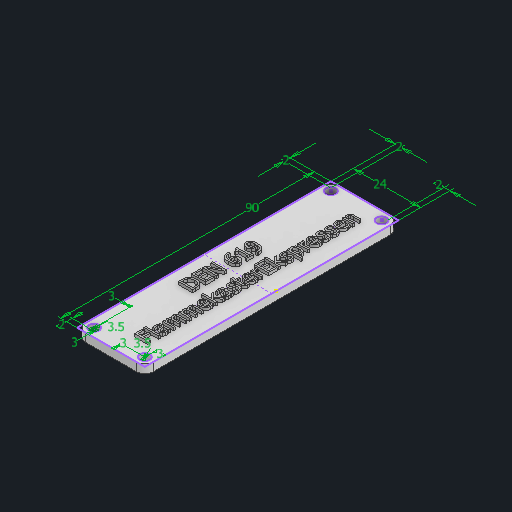
# Autodesk Inventor part: Flammekasterekspressen
Saved by Autodesk Inventor 2026.2 (Build 302298000, 298)
## iProperties
Created: 2026-05-12
Part Number: Flammekasterekspressen
Material: Generic
Document SubType Name: Modeling
Designer: Malthe Sennels
Density: 1 g/cm^3
Appearance: Default
Author: Malthe Sennels
Autodesk Inventor part; units mm, degrees
ref_plane "YZ Plane" through (0, 0, 0) normal (1, 0, 0) x (0, 1, 0)
ref_plane "XZ Plane" through (0, 0, 0) normal (0, 1, 0) x (-1, 0, 0)
ref_plane "XY Plane" through (0, 0, 0) normal (0, 0, 1) x (1, 0, 0)
sketch "Sketch1" plane through (0, 0, 0) normal (0, 1, 0) x (-1, 0, 0)
  line L0 (24.0563, 46.4821) -> (0.0563, 46.4821)
  line L1 (0.0563, 46.4821) -> (0.0563, -43.5179)
  line L2 (0.0563, -43.5179) -> (24.0563, -43.5179)
  line L3 (24.0563, -43.5179) -> (24.0563, 46.4821)
  line L4 (22.0563, 44.4821) -> (22.0563, -41.5179) construction
  line L5 (22.0563, -41.5179) -> (2.0563, -41.5179) construction
  line L6 (2.0563, -41.5179) -> (2.0563, 44.4821) construction
  line L7 (2.0563, 44.4821) -> (22.0563, 44.4821) construction
  circle A0 centre (21.0563, 43.4821) radius 1.75
  circle A1 centre (3.0563, 43.4821) radius 1.75
  line L8 (24.0563, 1.4821) -> (0.0563, 1.4821) construction
  circle A2 centre (21.0563, -40.5179) radius 1.75
  circle A3 centre (3.0563, -40.5179) radius 1.75
  spline S0 degree 2 poles (16.8086, 11.3646) (16.1238, 11.3646) (15.0217, 11.9197) (14.7138, 12.3857) knots 0 0 0 1 2 2 2
  spline S1 degree 2 poles (14.7138, 12.3857) (14.4747, 12.7666) (14.3126, 13.5486) (14.3126, 14.1564) knots 0 0 0 1 2 2 2
  line L9 (14.3126, 14.1564) -> (14.3126, 15.3071)
  line L10 (14.3126, 15.3071) -> (19.3126, 15.3071)
  line L11 (19.3126, 15.3071) -> (19.3126, 14.1685)
  spline S2 degree 2 poles (19.3126, 14.1685) (19.3126, 13.4635) (19.1019, 12.6612) (18.9156, 12.3776) knots 0 0 0 1 2 2 2
  spline S3 degree 2 poles (18.9156, 12.3776) (18.5955, 11.8954) (17.5379, 11.3646) (16.8086, 11.3646) knots 0 0 0 1 2 2 2
  spline S4 degree 2 poles (16.8167, 12.0575) (17.3921, 12.0575) (18.2065, 12.4384) (18.4374, 12.8152) knots 0 0 0 1 2 2 2
  spline S5 degree 2 poles (18.4374, 12.8152) (18.5955, 13.0826) (18.7373, 13.6863) (18.7373, 14.1361) knots 0 0 0 1 2 2 2
  line L12 (18.7373, 14.1361) -> (18.7373, 14.6426)
  line L13 (18.7373, 14.6426) -> (14.888, 14.6426)
  line L14 (14.888, 14.6426) -> (14.888, 14.1361)
  spline S6 degree 2 poles (14.888, 14.1361) (14.888, 13.6945) (15.0298, 13.0259) (15.2203, 12.7544) knots 0 0 0 1 2 2 2
  spline S7 degree 2 poles (15.2203, 12.7544) (15.4553, 12.406) (16.2332, 12.0575) (16.8167, 12.0575) knots 0 0 0 1 2 2 2
  line L15 (14.3126, 10.6434) -> (19.3126, 10.6434)
  line L16 (19.3126, 10.6434) -> (19.3126, 7.5154)
  line L17 (19.3126, 7.5154) -> (18.7211, 7.5154)
  line L18 (18.7211, 7.5154) -> (18.7211, 9.9789)
  line L19 (18.7211, 9.9789) -> (17.3515, 9.9789)
  line L20 (17.3515, 9.9789) -> (17.3515, 7.6815)
  line L21 (17.3515, 7.6815) -> (16.76, 7.6815)
  line L22 (16.76, 7.6815) -> (16.76, 9.9789)
  line L23 (16.76, 9.9789) -> (14.9042, 9.9789)
  line L24 (14.9042, 9.9789) -> (14.9042, 7.5154)
  line L25 (14.9042, 7.5154) -> (14.3126, 7.5154)
  line L26 (14.3126, 7.5154) -> (14.3126, 10.6434)
  line L27 (14.3126, 3.2082) -> (14.3126, 3.9538)
  line L28 (14.3126, 3.9538) -> (18.6238, 6.1661)
  line L29 (18.6238, 6.1661) -> (14.3126, 6.1661)
  line L30 (14.3126, 6.1661) -> (14.3126, 6.786)
  line L31 (14.3126, 6.786) -> (19.3126, 6.786)
  line L32 (19.3126, 6.786) -> (19.3126, 5.8419)
  line L33 (19.3126, 5.8419) -> (15.354, 3.8282)
  line L34 (15.354, 3.8282) -> (19.3126, 3.8282)
  line L35 (19.3126, 3.8282) -> (19.3126, 3.2082)
  line L36 (19.3126, 3.2082) -> (14.3126, 3.2082)
  spline S8 degree 2 poles (15.9334, -2.9709) (15.5485, -2.9709) (14.8961, -2.7156) (14.6773, -2.5008) knots 0 0 0 1 2 2 2
  spline S9 degree 2 poles (14.6773, -2.5008) (14.4464, -2.278) (14.2073, -1.7188) (14.2073, -1.3825) knots 0 0 0 1 2 2 2
  spline S10 degree 2 poles (14.2073, -1.3825) (14.2073, -1.0462) (14.4342, -0.4911) (14.6611, -0.2804) knots 0 0 0 1 2 2 2
  spline S11 degree 2 poles (14.6611, -0.2804) (14.9326, -0.0211) (15.8443, 0.2706) (16.5088, 0.2706) knots 0 0 0 1 2 2 2
  spline S12 degree 2 poles (16.5088, 0.2706) (17.1611, 0.2706) (18.2105, 0.0032) (18.5995, -0.2764) knots 0 0 0 1 2 2 2
  spline S13 degree 2 poles (18.5995, -0.2764) (18.9804, -0.5478) (19.4058, -1.4068) (19.4058, -1.9701) knots 0 0 0 1 2 2 2
  spline S14 degree 2 poles (19.4058, -1.9701) (19.4058, -2.1362) (19.3734, -2.4279) (19.337, -2.5373) knots 0 0 0 1 2 2 2
  line L37 (19.337, -2.5373) -> (18.6927, -2.5373)
  line L38 (18.6927, -2.5373) -> (18.6927, -2.509)
  spline S15 degree 2 poles (18.6927, -2.509) (18.7413, -2.4158) (18.8264, -2.0754) (18.8264, -1.8809) knots 0 0 0 1 2 2 2
  spline S16 degree 2 poles (18.8264, -1.8809) (18.8264, -1.2569) (17.9836, -0.4911) (17.1571, -0.4182) knots 0 0 0 1 2 2 2
  spline S17 degree 2 poles (17.1571, -0.4182) (17.3232, -0.6572) (17.5055, -1.1597) (17.5055, -1.4595) knots 0 0 0 1 2 2 2
  spline S18 degree 2 poles (17.5055, -1.4595) (17.5055, -1.7513) (17.388, -2.1889) (17.2097, -2.4279) knots 0 0 0 1 2 2 2
  spline S19 degree 2 poles (17.2097, -2.4279) (17.0031, -2.7034) (16.3629, -2.9709) (15.9334, -2.9709) knots 0 0 0 1 2 2 2
  spline S20 degree 2 poles (15.905, -2.2902) (16.213, -2.2902) (16.6303, -2.1281) (16.7762, -1.9498) knots 0 0 0 1 2 2 2
  spline S21 degree 2 poles (16.7762, -1.9498) (16.8815, -1.8161) (16.9504, -1.4838) (16.9504, -1.3096) knots 0 0 0 1 2 2 2
  spline S22 degree 2 poles (16.9504, -1.3096) (16.9504, -1.0746) (16.8086, -0.6329) (16.6749, -0.4182) knots 0 0 0 1 2 2 2
  spline S23 degree 2 poles (16.6749, -0.4182) (16.6019, -0.4141) (16.4642, -0.406) (16.3588, -0.406) knots 0 0 0 1 2 2 2
  spline S24 degree 2 poles (16.3588, -0.406) (15.8402, -0.406) (15.2041, -0.6086) (15.0379, -0.7626) knots 0 0 0 1 2 2 2
  spline S25 degree 2 poles (15.0379, -0.7626) (14.8799, -0.9044) (14.7543, -1.2124) (14.7543, -1.3866) knots 0 0 0 1 2 2 2
  spline S26 degree 2 poles (14.7543, -1.3866) (14.7543, -1.7918) (15.3297, -2.2902) (15.905, -2.2902) knots 0 0 0 1 2 2 2
  line L39 (14.3126, -6.3947) -> (14.3126, -3.9555)
  line L40 (14.3126, -3.9555) -> (14.8232, -3.9555)
  line L41 (14.8232, -3.9555) -> (14.8232, -4.8631)
  line L42 (14.8232, -4.8631) -> (18.1741, -4.8631)
  line L43 (18.1741, -4.8631) -> (18.1741, -3.9555)
  line L44 (18.1741, -3.9555) -> (18.6319, -3.9555)
  spline S27 degree 2 poles (18.6319, -3.9555) (18.6319, -4.4701) (18.9237, -4.9563) (19.3289, -4.9887) knots 0 0 0 1 2 2 2
  line L45 (19.3289, -4.9887) -> (19.3289, -5.5073)
  line L46 (19.3289, -5.5073) -> (14.8232, -5.5073)
  line L47 (14.8232, -5.5073) -> (14.8232, -6.3947)
  line L48 (14.8232, -6.3947) -> (14.3126, -6.3947)
  spline S28 degree 2 poles (17.6878, -7.1767) (18.0728, -7.1767) (18.713, -7.4279) (18.9439, -7.6467) knots 0 0 0 1 2 2 2
  spline S29 degree 2 poles (18.9439, -7.6467) (19.1668, -7.8534) (19.4139, -8.4571) (19.4139, -8.765) knots 0 0 0 1 2 2 2
  spline S30 degree 2 poles (19.4139, -8.765) (19.4139, -9.1094) (19.183, -9.6686) (18.9642, -9.8752) knots 0 0 0 1 2 2 2
  spline S31 degree 2 poles (18.9642, -9.8752) (18.6887, -10.1346) (17.7972, -10.4182) (17.1125, -10.4182) knots 0 0 0 1 2 2 2
  spline S32 degree 2 poles (17.1125, -10.4182) (16.4925, -10.4182) (15.3823, -10.1386) (15.0136, -9.8671) knots 0 0 0 1 2 2 2
  spline S33 degree 2 poles (15.0136, -9.8671) (14.6246, -9.5795) (14.2154, -8.7691) (14.2154, -8.1775) knots 0 0 0 1 2 2 2
  spline S34 degree 2 poles (14.2154, -8.1775) (14.2154, -8.0438) (14.2438, -7.7399) (14.2843, -7.6102) knots 0 0 0 1 2 2 2
  line L49 (14.2843, -7.6102) -> (14.9285, -7.6102)
  line L50 (14.9285, -7.6102) -> (14.9285, -7.6427)
  spline S35 degree 2 poles (14.9285, -7.6427) (14.8799, -7.7278) (14.7948, -8.0843) (14.7948, -8.2666) knots 0 0 0 1 2 2 2
  spline S36 degree 2 poles (14.7948, -8.2666) (14.7948, -8.9231) (15.6619, -9.6726) (16.4642, -9.7253) knots 0 0 0 1 2 2 2
  spline S37 degree 2 poles (16.4642, -9.7253) (16.2819, -9.4579) (16.1157, -8.9717) (16.1157, -8.684) knots 0 0 0 1 2 2 2
  spline S38 degree 2 poles (16.1157, -8.684) (16.1157, -8.4085) (16.2373, -7.9506) (16.4115, -7.7196) knots 0 0 0 1 2 2 2
  spline S39 degree 2 poles (16.4115, -7.7196) (16.6182, -7.4522) (17.2462, -7.1767) (17.6878, -7.1767) knots 0 0 0 1 2 2 2
  spline S40 degree 2 poles (17.2624, -9.7415) (17.7689, -9.7415) (18.4091, -9.5551) (18.5833, -9.389) knots 0 0 0 1 2 2 2
  spline S41 degree 2 poles (18.5833, -9.389) (18.7454, -9.2431) (18.8669, -8.9393) (18.8669, -8.761) knots 0 0 0 1 2 2 2
  spline S42 degree 2 poles (18.8669, -8.761) (18.8669, -8.3477) (18.2754, -7.8574) (17.7162, -7.8574) knots 0 0 0 1 2 2 2
  spline S43 degree 2 poles (17.7162, -7.8574) (17.4002, -7.8574) (16.9909, -8.0195) (16.8451, -8.1978) knots 0 0 0 1 2 2 2
  spline S44 degree 2 poles (16.8451, -8.1978) (16.7397, -8.3274) (16.6708, -8.6475) (16.6708, -8.8339) knots 0 0 0 1 2 2 2
  spline S45 degree 2 poles (16.6708, -8.8339) (16.6708, -9.0487) (16.8207, -9.543) (16.9464, -9.7294) knots 0 0 0 1 2 2 2
  spline S46 degree 2 poles (16.9464, -9.7294) (16.995, -9.7334) (17.1611, -9.7415) (17.2624, -9.7415) knots 0 0 0 1 2 2 2
  line L51 (10.4887, 36.1195) -> (10.4887, 38.4453)
  line L52 (10.4887, 38.4453) -> (9.0787, 38.4453)
  line L53 (9.0787, 38.4453) -> (9.0787, 36.2167)
  line L54 (9.0787, 36.2167) -> (8.4871, 36.2167)
  line L55 (8.4871, 36.2167) -> (8.4871, 38.4453)
  line L56 (8.4871, 38.4453) -> (6.0803, 38.4453)
  line L57 (6.0803, 38.4453) -> (6.0803, 39.1098)
  line L58 (6.0803, 39.1098) -> (11.0803, 39.1098)
  line L59 (11.0803, 39.1098) -> (11.0803, 36.1195)
  line L60 (11.0803, 36.1195) -> (10.4887, 36.1195)
  line L61 (6.0803, 34.9282) -> (6.0803, 35.5603)
  line L62 (6.0803, 35.5603) -> (11.3031, 35.5603)
  line L63 (11.3031, 35.5603) -> (11.3031, 34.9282)
  line L64 (11.3031, 34.9282) -> (6.0803, 34.9282)
  spline S47 degree 2 poles (6.4774, 31.9096) (6.4206, 31.9866) (6.218, 32.2459) (6.1573, 32.3675) knots 0 0 0 1 2 2 2
  spline S48 degree 2 poles (6.1573, 32.3675) (6.0681, 32.5336) (5.9749, 32.8456) (5.9749, 33.1292) knots 0 0 0 1 2 2 2
  spline S49 degree 2 poles (5.9749, 33.1292) (5.9749, 33.3602) (6.1492, 33.7775) (6.3072, 33.9355) knots 0 0 0 1 2 2 2
  spline S50 degree 2 poles (6.3072, 33.9355) (6.4612, 34.0855) (6.915, 34.2678) (7.1662, 34.2678) knots 0 0 0 1 2 2 2
  spline S51 degree 2 poles (7.1662, 34.2678) (7.5552, 34.2678) (8.1062, 33.9396) (8.2642, 33.583) knots 0 0 0 1 2 2 2
  spline S52 degree 2 poles (8.2642, 33.583) (8.4101, 33.267) (8.5195, 32.408) (8.5479, 31.9096) knots 0 0 0 1 2 2 2
  line L65 (8.5479, 31.9096) -> (8.6694, 31.9096)
  spline S53 degree 2 poles (8.6694, 31.9096) (8.8882, 31.9096) (9.1597, 32.0433) (9.2367, 32.1649) knots 0 0 0 1 2 2 2
  spline S54 degree 2 poles (9.2367, 32.1649) (9.3137, 32.2864) (9.3623, 32.6349) (9.3623, 32.8213) knots 0 0 0 1 2 2 2
  spline S55 degree 2 poles (9.3623, 32.8213) (9.3623, 33.0401) (9.2326, 33.6316) (9.107, 33.9274) knots 0 0 0 1 2 2 2
  line L66 (9.107, 33.9274) -> (9.107, 33.9639)
  line L67 (9.107, 33.9639) -> (9.7513, 33.9639)
  spline S56 degree 2 poles (9.7513, 33.9639) (9.7999, 33.7897) (9.9214, 33.1373) (9.9214, 32.8172) knots 0 0 0 1 2 2 2
  spline S57 degree 2 poles (9.9214, 32.8172) (9.9214, 32.4282) (9.7999, 31.8975) (9.6419, 31.6868) knots 0 0 0 1 2 2 2
  spline S58 degree 2 poles (9.6419, 31.6868) (9.4879, 31.4801) (8.9976, 31.2775) (8.6451, 31.2775) knots 0 0 0 1 2 2 2
  line L68 (8.6451, 31.2775) -> (6.0803, 31.2775)
  line L69 (6.0803, 31.2775) -> (6.0803, 31.9096)
  line L70 (6.0803, 31.9096) -> (6.4774, 31.9096)
  line L71 (7.0041, 31.9096) -> (8.0454, 31.9096)
  spline S59 degree 2 poles (8.0454, 31.9096) (8.0252, 32.1365) (7.9563, 32.8213) (7.8915, 33.036) knots 0 0 0 1 2 2 2
  spline S60 degree 2 poles (7.8915, 33.036) (7.8145, 33.2872) (7.4944, 33.6154) (7.2107, 33.6154) knots 0 0 0 1 2 2 2
  spline S61 degree 2 poles (7.2107, 33.6154) (6.8866, 33.6154) (6.5584, 33.2508) (6.5584, 32.9023) knots 0 0 0 1 2 2 2
  spline S62 degree 2 poles (6.5584, 32.9023) (6.5584, 32.6065) (6.8137, 32.1203) (7.0041, 31.9096) knots 0 0 0 1 2 2 2
  line L72 (6.0803, 26.1357) -> (8.2521, 26.1357)
  spline S63 degree 2 poles (8.2521, 26.1357) (8.5114, 26.1357) (8.953, 26.1762) (9.0746, 26.241) knots 0 0 0 1 2 2 2
  spline S64 degree 2 poles (9.0746, 26.241) (9.2083, 26.3059) (9.338, 26.553) (9.338, 26.7678) knots 0 0 0 1 2 2 2
  spline S65 degree 2 poles (9.338, 26.7678) (9.338, 26.9623) (9.0989, 27.408) (8.872, 27.643) knots 0 0 0 1 2 2 2
  spline S66 degree 2 poles (8.872, 27.643) (8.8153, 27.6389) (8.6573, 27.6308) (8.5519, 27.6308) knots 0 0 0 1 2 2 2
  line L73 (8.5519, 27.6308) -> (6.0803, 27.6308)
  line L74 (6.0803, 27.6308) -> (6.0803, 28.2629)
  line L75 (6.0803, 28.2629) -> (8.2521, 28.2629)
  spline S67 degree 2 poles (8.2521, 28.2629) (8.5114, 28.2629) (8.953, 28.3034) (9.0746, 28.3683) knots 0 0 0 1 2 2 2
  spline S68 degree 2 poles (9.0746, 28.3683) (9.2083, 28.4331) (9.338, 28.6803) (9.338, 28.895) knots 0 0 0 1 2 2 2
  spline S69 degree 2 poles (9.338, 28.895) (9.338, 29.0976) (9.0827, 29.5474) (8.8842, 29.7581) knots 0 0 0 1 2 2 2
  line L76 (8.8842, 29.7581) -> (6.0803, 29.7581)
  line L77 (6.0803, 29.7581) -> (6.0803, 30.3902)
  line L78 (6.0803, 30.3902) -> (9.8323, 30.3902)
  line L79 (9.8323, 30.3902) -> (9.8323, 29.7581)
  line L80 (9.8323, 29.7581) -> (9.419, 29.7581)
  spline S70 degree 2 poles (9.419, 29.7581) (9.6662, 29.5109) (9.9377, 29.0247) (9.9377, 28.7329) knots 0 0 0 1 2 2 2
  spline S71 degree 2 poles (9.9377, 28.7329) (9.9377, 28.4007) (9.6338, 27.8861) (9.2894, 27.7524) knots 0 0 0 1 2 2 2
  spline S72 degree 2 poles (9.2894, 27.7524) (9.6095, 27.4647) (9.9377, 26.9218) (9.9377, 26.6057) knots 0 0 0 1 2 2 2
  spline S73 degree 2 poles (9.9377, 26.6057) (9.9377, 26.3626) (9.7877, 25.9655) (9.6176, 25.8197) knots 0 0 0 1 2 2 2
  spline S74 degree 2 poles (9.6176, 25.8197) (9.4474, 25.6697) (8.9368, 25.5036) (8.5519, 25.5036) knots 0 0 0 1 2 2 2
  line L81 (8.5519, 25.5036) -> (6.0803, 25.5036)
  line L82 (6.0803, 25.5036) -> (6.0803, 26.1357)
  line L83 (6.0803, 20.3618) -> (8.2521, 20.3618)
  spline S75 degree 2 poles (8.2521, 20.3618) (8.5114, 20.3618) (8.953, 20.4023) (9.0746, 20.4671) knots 0 0 0 1 2 2 2
  spline S76 degree 2 poles (9.0746, 20.4671) (9.2083, 20.532) (9.338, 20.7791) (9.338, 20.9939) knots 0 0 0 1 2 2 2
  spline S77 degree 2 poles (9.338, 20.9939) (9.338, 21.1884) (9.0989, 21.6341) (8.872, 21.8691) knots 0 0 0 1 2 2 2
  spline S78 degree 2 poles (8.872, 21.8691) (8.8153, 21.865) (8.6573, 21.8569) (8.5519, 21.8569) knots 0 0 0 1 2 2 2
  line L84 (8.5519, 21.8569) -> (6.0803, 21.8569)
  line L85 (6.0803, 21.8569) -> (6.0803, 22.489)
  line L86 (6.0803, 22.489) -> (8.2521, 22.489)
  spline S79 degree 2 poles (8.2521, 22.489) (8.5114, 22.489) (8.953, 22.5295) (9.0746, 22.5944) knots 0 0 0 1 2 2 2
  spline S80 degree 2 poles (9.0746, 22.5944) (9.2083, 22.6592) (9.338, 22.9064) (9.338, 23.1211) knots 0 0 0 1 2 2 2
  spline S81 degree 2 poles (9.338, 23.1211) (9.338, 23.3237) (9.0827, 23.7735) (8.8842, 23.9842) knots 0 0 0 1 2 2 2
  line L87 (8.8842, 23.9842) -> (6.0803, 23.9842)
  line L88 (6.0803, 23.9842) -> (6.0803, 24.6163)
  line L89 (6.0803, 24.6163) -> (9.8323, 24.6163)
  line L90 (9.8323, 24.6163) -> (9.8323, 23.9842)
  line L91 (9.8323, 23.9842) -> (9.419, 23.9842)
  spline S82 degree 2 poles (9.419, 23.9842) (9.6662, 23.737) (9.9377, 23.2508) (9.9377, 22.959) knots 0 0 0 1 2 2 2
  spline S83 degree 2 poles (9.9377, 22.959) (9.9377, 22.6268) (9.6338, 22.1122) (9.2894, 21.9785) knots 0 0 0 1 2 2 2
  spline S84 degree 2 poles (9.2894, 21.9785) (9.6095, 21.6908) (9.9377, 21.1479) (9.9377, 20.8318) knots 0 0 0 1 2 2 2
  spline S85 degree 2 poles (9.9377, 20.8318) (9.9377, 20.5887) (9.7877, 20.1916) (9.6176, 20.0457) knots 0 0 0 1 2 2 2
  spline S86 degree 2 poles (9.6176, 20.0457) (9.4474, 19.8958) (8.9368, 19.7297) (8.5519, 19.7297) knots 0 0 0 1 2 2 2
  line L92 (8.5519, 19.7297) -> (6.0803, 19.7297)
  line L93 (6.0803, 19.7297) -> (6.0803, 20.3618)
  spline S87 degree 2 poles (5.9952, 17.2135) (5.9952, 18.113) (7.0041, 19.1017) (7.936, 19.1017) knots 0 0 0 1 2 2 2
  spline S88 degree 2 poles (7.936, 19.1017) (8.8518, 19.1017) (9.9377, 18.1414) (9.9377, 17.3675) knots 0 0 0 1 2 2 2
  spline S89 degree 2 poles (9.9377, 17.3675) (9.9377, 17.019) (9.7351, 16.4801) (9.5203, 16.2816) knots 0 0 0 1 2 2 2
  spline S90 degree 2 poles (9.5203, 16.2816) (9.3056, 16.079) (8.6856, 15.8642) (8.2359, 15.8642) knots 0 0 0 1 2 2 2
  line L94 (8.2359, 15.8642) -> (7.8915, 15.8642)
  line L95 (7.8915, 15.8642) -> (7.8915, 18.4615)
  spline S91 degree 2 poles (7.8915, 18.4615) (7.2391, 18.4615) (6.5462, 17.8051) (6.5462, 17.2216) knots 0 0 0 1 2 2 2
  spline S92 degree 2 poles (6.5462, 17.2216) (6.5462, 17.015) (6.6394, 16.6138) (6.7124, 16.4517) knots 0 0 0 1 2 2 2
  spline S93 degree 2 poles (6.7124, 16.4517) (6.7934, 16.2816) (6.9352, 16.0466) (7.0001, 15.9696) knots 0 0 0 1 2 2 2
  line L96 (7.0001, 15.9696) -> (7.0001, 15.9331)
  line L97 (7.0001, 15.9331) -> (6.3112, 15.9331)
  spline S94 degree 2 poles (6.3112, 15.9331) (6.2667, 16.0425) (6.137, 16.3748) (6.1005, 16.5044) knots 0 0 0 1 2 2 2
  spline S95 degree 2 poles (6.1005, 16.5044) (6.0479, 16.6868) (5.9952, 16.9866) (5.9952, 17.2135) knots 0 0 0 1 2 2 2
  spline S96 degree 2 poles (8.3736, 16.4801) (8.6289, 16.4882) (9.0017, 16.5936) (9.1273, 16.6949) knots 0 0 0 1 2 2 2
  spline S97 degree 2 poles (9.1273, 16.6949) (9.2691, 16.8043) (9.419, 17.1487) (9.419, 17.4039) knots 0 0 0 1 2 2 2
  spline S98 degree 2 poles (9.419, 17.4039) (9.419, 17.6551) (9.2691, 18.0077) (9.1232, 18.1535) knots 0 0 0 1 2 2 2
  spline S99 degree 2 poles (9.1232, 18.1535) (8.9733, 18.2953) (8.6127, 18.4412) (8.3736, 18.4615) knots 0 0 0 1 2 2 2
  line L98 (8.3736, 18.4615) -> (8.3736, 16.4801)
  line L99 (6.0803, 12.1163) -> (6.0803, 12.9469)
  line L100 (6.0803, 12.9469) -> (7.8915, 14.3407)
  line L101 (7.8915, 14.3407) -> (7.6483, 14.5919)
  line L102 (7.6483, 14.5919) -> (6.0803, 14.5919)
  line L103 (6.0803, 14.5919) -> (6.0803, 15.224)
  line L104 (6.0803, 15.224) -> (11.3031, 15.224)
  line L105 (11.3031, 15.224) -> (11.3031, 14.5919)
  line L106 (11.3031, 14.5919) -> (8.248, 14.5919)
  line L107 (8.248, 14.5919) -> (9.8323, 13.109)
  line L108 (9.8323, 13.109) -> (9.8323, 12.3229)
  line L109 (9.8323, 12.3229) -> (8.2642, 13.8626)
  line L110 (8.2642, 13.8626) -> (6.0803, 12.1163)
  spline S100 degree 2 poles (6.4774, 9.7094) (6.4206, 9.7864) (6.218, 10.0457) (6.1573, 10.1673) knots 0 0 0 1 2 2 2
  spline S101 degree 2 poles (6.1573, 10.1673) (6.0681, 10.3334) (5.9749, 10.6454) (5.9749, 10.9291) knots 0 0 0 1 2 2 2
  spline S102 degree 2 poles (5.9749, 10.9291) (5.9749, 11.16) (6.1492, 11.5774) (6.3072, 11.7354) knots 0 0 0 1 2 2 2
  spline S103 degree 2 poles (6.3072, 11.7354) (6.4612, 11.8853) (6.915, 12.0676) (7.1662, 12.0676) knots 0 0 0 1 2 2 2
  spline S104 degree 2 poles (7.1662, 12.0676) (7.5552, 12.0676) (8.1062, 11.7394) (8.2642, 11.3829) knots 0 0 0 1 2 2 2
  spline S105 degree 2 poles (8.2642, 11.3829) (8.4101, 11.0668) (8.5195, 10.2078) (8.5479, 9.7094) knots 0 0 0 1 2 2 2
  line L111 (8.5479, 9.7094) -> (8.6694, 9.7094)
  spline S106 degree 2 poles (8.6694, 9.7094) (8.8882, 9.7094) (9.1597, 9.8432) (9.2367, 9.9647) knots 0 0 0 1 2 2 2
  spline S107 degree 2 poles (9.2367, 9.9647) (9.3137, 10.0863) (9.3623, 10.4347) (9.3623, 10.6211) knots 0 0 0 1 2 2 2
  spline S108 degree 2 poles (9.3623, 10.6211) (9.3623, 10.8399) (9.2326, 11.4315) (9.107, 11.7273) knots 0 0 0 1 2 2 2
  line L112 (9.107, 11.7273) -> (9.107, 11.7637)
  line L113 (9.107, 11.7637) -> (9.7513, 11.7637)
  spline S109 degree 2 poles (9.7513, 11.7637) (9.7999, 11.5895) (9.9214, 10.9372) (9.9214, 10.6171) knots 0 0 0 1 2 2 2
  spline S110 degree 2 poles (9.9214, 10.6171) (9.9214, 10.2281) (9.7999, 9.6973) (9.6419, 9.4866) knots 0 0 0 1 2 2 2
  spline S111 degree 2 poles (9.6419, 9.4866) (9.4879, 9.2799) (8.9976, 9.0774) (8.6451, 9.0774) knots 0 0 0 1 2 2 2
  line L114 (8.6451, 9.0774) -> (6.0803, 9.0774)
  line L115 (6.0803, 9.0774) -> (6.0803, 9.7094)
  line L116 (6.0803, 9.7094) -> (6.4774, 9.7094)
  line L117 (7.0041, 9.7094) -> (8.0454, 9.7094)
  spline S112 degree 2 poles (8.0454, 9.7094) (8.0252, 9.9363) (7.9563, 10.6211) (7.8915, 10.8359) knots 0 0 0 1 2 2 2
  spline S113 degree 2 poles (7.8915, 10.8359) (7.8145, 11.0871) (7.4944, 11.4153) (7.2107, 11.4153) knots 0 0 0 1 2 2 2
  spline S114 degree 2 poles (7.2107, 11.4153) (6.8866, 11.4153) (6.5584, 11.0506) (6.5584, 10.7022) knots 0 0 0 1 2 2 2
  spline S115 degree 2 poles (6.5584, 10.7022) (6.5584, 10.4064) (6.8137, 9.9201) (7.0041, 9.7094) knots 0 0 0 1 2 2 2
  spline S116 degree 2 poles (5.9911, 7.177) (5.9911, 7.5539) (6.1937, 8.2062) (6.3072, 8.421) knots 0 0 0 1 2 2 2
  line L118 (6.3072, 8.421) -> (7.0163, 8.421)
  line L119 (7.0163, 8.421) -> (7.0163, 8.3885)
  spline S117 degree 2 poles (7.0163, 8.3885) (6.9514, 8.3075) (6.7975, 8.0887) (6.7124, 7.9064) knots 0 0 0 1 2 2 2
  spline S118 degree 2 poles (6.7124, 7.9064) (6.6354, 7.7483) (6.5219, 7.3594) (6.5219, 7.1527) knots 0 0 0 1 2 2 2
  spline S119 degree 2 poles (6.5219, 7.1527) (6.5219, 7.0028) (6.5908, 6.6584) (6.6475, 6.5774) knots 0 0 0 1 2 2 2
  spline S120 degree 2 poles (6.6475, 6.5774) (6.7245, 6.4599) (6.8988, 6.3545) (7.077, 6.3545) knots 0 0 0 1 2 2 2
  spline S121 degree 2 poles (7.077, 6.3545) (7.2999, 6.3545) (7.5308, 6.5976) (7.6078, 6.9096) knots 0 0 0 1 2 2 2
  spline S122 degree 2 poles (7.6078, 6.9096) (7.6362, 7.0312) (7.7172, 7.4201) (7.7618, 7.5863) knots 0 0 0 1 2 2 2
  spline S123 degree 2 poles (7.7618, 7.5863) (7.8874, 8.0158) (8.406, 8.4047) (8.7748, 8.4047) knots 0 0 0 1 2 2 2
  spline S124 degree 2 poles (8.7748, 8.4047) (9.2853, 8.4047) (9.9214, 7.6389) (9.9214, 7.0069) knots 0 0 0 1 2 2 2
  spline S125 degree 2 poles (9.9214, 7.0069) (9.9214, 6.6949) (9.7675, 6.0628) (9.65, 5.848) knots 0 0 0 1 2 2 2
  line L120 (9.65, 5.848) -> (8.9733, 5.848)
  line L121 (8.9733, 5.848) -> (8.9733, 5.8804)
  spline S126 degree 2 poles (8.9733, 5.8804) (9.1678, 6.1235) (9.3907, 6.7151) (9.3907, 7.019) knots 0 0 0 1 2 2 2
  spline S127 degree 2 poles (9.3907, 7.019) (9.3907, 7.331) (9.1273, 7.7605) (8.8639, 7.7605) knots 0 0 0 1 2 2 2
  spline S128 degree 2 poles (8.8639, 7.7605) (8.6248, 7.7605) (8.3939, 7.5052) (8.321, 7.2216) knots 0 0 0 1 2 2 2
  spline S129 degree 2 poles (8.321, 7.2216) (8.2845, 7.0838) (8.2116, 6.7354) (8.167, 6.5449) knots 0 0 0 1 2 2 2
  spline S130 degree 2 poles (8.167, 6.5449) (8.0616, 6.1316) (7.5795, 5.7103) (7.1621, 5.7103) knots 0 0 0 1 2 2 2
  spline S131 degree 2 poles (7.1621, 5.7103) (6.919, 5.7103) (6.4895, 5.9007) (6.3315, 6.0871) knots 0 0 0 1 2 2 2
  spline S132 degree 2 poles (6.3315, 6.0871) (6.1654, 6.2856) (5.9911, 6.7921) (5.9911, 7.177) knots 0 0 0 1 2 2 2
  spline S133 degree 2 poles (6.0073, 3.9882) (6.0073, 4.5028) (6.5949, 5.0822) (7.231, 5.0822) knots 0 0 0 1 2 2 2
  line L122 (7.231, 5.0822) -> (9.3096, 5.0822)
  line L123 (9.3096, 5.0822) -> (9.3096, 5.5077)
  line L124 (9.3096, 5.5077) -> (9.8323, 5.5077)
  line L125 (9.8323, 5.5077) -> (9.8323, 5.0822)
  line L126 (9.8323, 5.0822) -> (10.9101, 5.0822)
  line L127 (10.9101, 5.0822) -> (10.9101, 4.4501)
  line L128 (10.9101, 4.4501) -> (9.8323, 4.4501)
  line L129 (9.8323, 4.4501) -> (9.8323, 3.2872)
  line L130 (9.8323, 3.2872) -> (9.3096, 3.2872)
  line L131 (9.3096, 3.2872) -> (9.3096, 4.4501)
  line L132 (9.3096, 4.4501) -> (7.5227, 4.4501)
  spline S134 degree 2 poles (7.5227, 4.4501) (7.2391, 4.4501) (6.9271, 4.4299) (6.7934, 4.361) knots 0 0 0 1 2 2 2
  spline S135 degree 2 poles (6.7934, 4.361) (6.6759, 4.3043) (6.5584, 4.049) (6.5584, 3.8302) knots 0 0 0 1 2 2 2
  spline S136 degree 2 poles (6.5584, 3.8302) (6.5584, 3.6762) (6.6516, 3.3885) (6.68, 3.3237) knots 0 0 0 1 2 2 2
  line L133 (6.68, 3.3237) -> (6.68, 3.2872)
  line L134 (6.68, 3.2872) -> (6.1127, 3.2872)
  spline S137 degree 2 poles (6.1127, 3.2872) (6.0641, 3.4655) (6.0073, 3.8302) (6.0073, 3.9882) knots 0 0 0 1 2 2 2
  spline S138 degree 2 poles (5.9952, 1.1924) (5.9952, 2.0919) (7.0041, 3.0806) (7.936, 3.0806) knots 0 0 0 1 2 2 2
  spline S139 degree 2 poles (7.936, 3.0806) (8.8518, 3.0806) (9.9377, 2.1203) (9.9377, 1.3464) knots 0 0 0 1 2 2 2
  spline S140 degree 2 poles (9.9377, 1.3464) (9.9377, 0.9979) (9.7351, 0.459) (9.5203, 0.2605) knots 0 0 0 1 2 2 2
  spline S141 degree 2 poles (9.5203, 0.2605) (9.3056, 0.0579) (8.6856, -0.1568) (8.2359, -0.1568) knots 0 0 0 1 2 2 2
  line L135 (8.2359, -0.1568) -> (7.8915, -0.1568)
  line L136 (7.8915, -0.1568) -> (7.8915, 2.4404)
  spline S142 degree 2 poles (7.8915, 2.4404) (7.2391, 2.4404) (6.5462, 1.784) (6.5462, 1.2005) knots 0 0 0 1 2 2 2
  spline S143 degree 2 poles (6.5462, 1.2005) (6.5462, 0.9939) (6.6394, 0.5928) (6.7124, 0.4307) knots 0 0 0 1 2 2 2
  spline S144 degree 2 poles (6.7124, 0.4307) (6.7934, 0.2605) (6.9352, 0.0255) (7.0001, -0.0515) knots 0 0 0 1 2 2 2
  line L137 (7.0001, -0.0515) -> (7.0001, -0.088)
  line L138 (7.0001, -0.088) -> (6.3112, -0.088)
  spline S145 degree 2 poles (6.3112, -0.088) (6.2667, 0.0214) (6.137, 0.3537) (6.1005, 0.4834) knots 0 0 0 1 2 2 2
  spline S146 degree 2 poles (6.1005, 0.4834) (6.0479, 0.6657) (5.9952, 0.9655) (5.9952, 1.1924) knots 0 0 0 1 2 2 2
  spline S147 degree 2 poles (8.3736, 0.459) (8.6289, 0.4671) (9.0017, 0.5725) (9.1273, 0.6738) knots 0 0 0 1 2 2 2
  spline S148 degree 2 poles (9.1273, 0.6738) (9.2691, 0.7832) (9.419, 1.1276) (9.419, 1.3829) knots 0 0 0 1 2 2 2
  spline S149 degree 2 poles (9.419, 1.3829) (9.419, 1.6341) (9.2691, 1.9866) (9.1232, 2.1325) knots 0 0 0 1 2 2 2
  spline S150 degree 2 poles (9.1232, 2.1325) (8.9733, 2.2743) (8.6127, 2.4201) (8.3736, 2.4404) knots 0 0 0 1 2 2 2
  line L139 (8.3736, 2.4404) -> (8.3736, 0.459)
  line L140 (9.1556, -2.7865) -> (9.1556, -2.7541)
  spline S151 degree 2 poles (9.1556, -2.7541) (9.1759, -2.6812) (9.184, -2.5231) (9.184, -2.4137) knots 0 0 0 1 2 2 2
  spline S152 degree 2 poles (9.184, -2.4137) (9.184, -2.1585) (8.9612, -1.656) (8.7424, -1.4291) knots 0 0 0 1 2 2 2
  line L141 (8.7424, -1.4291) -> (6.0803, -1.4291)
  line L142 (6.0803, -1.4291) -> (6.0803, -0.797)
  line L143 (6.0803, -0.797) -> (9.8323, -0.797)
  line L144 (9.8323, -0.797) -> (9.8323, -1.4291)
  line L145 (9.8323, -1.4291) -> (9.2731, -1.4291)
  spline S153 degree 2 poles (9.2731, -1.4291) (9.5811, -1.7735) (9.8323, -2.2881) (9.8323, -2.5312) knots 0 0 0 1 2 2 2
  spline S154 degree 2 poles (9.8323, -2.5312) (9.8323, -2.6285) (9.8242, -2.7257) (9.812, -2.7865) knots 0 0 0 1 2 2 2
  line L146 (9.812, -2.7865) -> (9.1556, -2.7865)
  line L147 (6.0803, -3.3254) -> (11.0803, -3.3254)
  line L148 (11.0803, -3.3254) -> (11.0803, -6.4534)
  line L149 (11.0803, -6.4534) -> (10.4887, -6.4534)
  line L150 (10.4887, -6.4534) -> (10.4887, -3.9899)
  line L151 (10.4887, -3.9899) -> (9.1192, -3.9899)
  line L152 (9.1192, -3.9899) -> (9.1192, -6.2873)
  line L153 (9.1192, -6.2873) -> (8.5276, -6.2873)
  line L154 (8.5276, -6.2873) -> (8.5276, -3.9899)
  line L155 (8.5276, -3.9899) -> (6.6719, -3.9899)
  line L156 (6.6719, -3.9899) -> (6.6719, -6.4534)
  line L157 (6.6719, -6.4534) -> (6.0803, -6.4534)
  line L158 (6.0803, -6.4534) -> (6.0803, -3.3254)
  line L159 (6.0803, -10.2419) -> (6.0803, -9.4113)
  line L160 (6.0803, -9.4113) -> (7.8915, -8.0175)
  line L161 (7.8915, -8.0175) -> (7.6483, -7.7662)
  line L162 (7.6483, -7.7662) -> (6.0803, -7.7662)
  line L163 (6.0803, -7.7662) -> (6.0803, -7.1342)
  line L164 (6.0803, -7.1342) -> (11.3031, -7.1342)
  line L165 (11.3031, -7.1342) -> (11.3031, -7.7662)
  line L166 (11.3031, -7.7662) -> (8.248, -7.7662)
  line L167 (8.248, -7.7662) -> (9.8323, -9.2492)
  line L168 (9.8323, -9.2492) -> (9.8323, -10.0353)
  line L169 (9.8323, -10.0353) -> (8.2642, -8.4956)
  line L170 (8.2642, -8.4956) -> (6.0803, -10.2419)
  spline S155 degree 2 poles (5.9911, -11.5709) (5.9911, -11.1941) (6.1937, -10.5418) (6.3072, -10.327) knots 0 0 0 1 2 2 2
  line L171 (6.3072, -10.327) -> (7.0163, -10.327)
  line L172 (7.0163, -10.327) -> (7.0163, -10.3594)
  spline S156 degree 2 poles (7.0163, -10.3594) (6.9514, -10.4405) (6.7975, -10.6593) (6.7124, -10.8416) knots 0 0 0 1 2 2 2
  spline S157 degree 2 poles (6.7124, -10.8416) (6.6354, -10.9996) (6.5219, -11.3886) (6.5219, -11.5953) knots 0 0 0 1 2 2 2
  spline S158 degree 2 poles (6.5219, -11.5953) (6.5219, -11.7452) (6.5908, -12.0896) (6.6475, -12.1706) knots 0 0 0 1 2 2 2
  spline S159 degree 2 poles (6.6475, -12.1706) (6.7245, -12.2881) (6.8988, -12.3935) (7.077, -12.3935) knots 0 0 0 1 2 2 2
  spline S160 degree 2 poles (7.077, -12.3935) (7.2999, -12.3935) (7.5308, -12.1504) (7.6078, -11.8384) knots 0 0 0 1 2 2 2
  spline S161 degree 2 poles (7.6078, -11.8384) (7.6362, -11.7168) (7.7172, -11.3278) (7.7618, -11.1617) knots 0 0 0 1 2 2 2
  spline S162 degree 2 poles (7.7618, -11.1617) (7.8874, -10.7322) (8.406, -10.3432) (8.7748, -10.3432) knots 0 0 0 1 2 2 2
  spline S163 degree 2 poles (8.7748, -10.3432) (9.2853, -10.3432) (9.9214, -11.109) (9.9214, -11.7411) knots 0 0 0 1 2 2 2
  spline S164 degree 2 poles (9.9214, -11.7411) (9.9214, -12.0531) (9.7675, -12.6852) (9.65, -12.9) knots 0 0 0 1 2 2 2
  line L173 (9.65, -12.9) -> (8.9733, -12.9)
  line L174 (8.9733, -12.9) -> (8.9733, -12.8675)
  spline S165 degree 2 poles (8.9733, -12.8675) (9.1678, -12.6244) (9.3907, -12.0329) (9.3907, -11.729) knots 0 0 0 1 2 2 2
  spline S166 degree 2 poles (9.3907, -11.729) (9.3907, -11.417) (9.1273, -10.9875) (8.8639, -10.9875) knots 0 0 0 1 2 2 2
  spline S167 degree 2 poles (8.8639, -10.9875) (8.6248, -10.9875) (8.3939, -11.2427) (8.321, -11.5264) knots 0 0 0 1 2 2 2
  spline S168 degree 2 poles (8.321, -11.5264) (8.2845, -11.6641) (8.2116, -12.0126) (8.167, -12.203) knots 0 0 0 1 2 2 2
  spline S169 degree 2 poles (8.167, -12.203) (8.0616, -12.6163) (7.5795, -13.0377) (7.1621, -13.0377) knots 0 0 0 1 2 2 2
  spline S170 degree 2 poles (7.1621, -13.0377) (6.919, -13.0377) (6.4895, -12.8473) (6.3315, -12.6609) knots 0 0 0 1 2 2 2
  spline S171 degree 2 poles (6.3315, -12.6609) (6.1654, -12.4624) (5.9911, -11.9559) (5.9911, -11.5709) knots 0 0 0 1 2 2 2
  spline S172 degree 2 poles (8.0576, -16.7695) (7.1176, -16.7695) (6.0073, -15.874) (6.0073, -15.1893) knots 0 0 0 1 2 2 2
  spline S173 degree 2 poles (6.0073, -15.1893) (6.0073, -14.9097) (6.137, -14.4802) (6.2707, -14.2573) knots 0 0 0 1 2 2 2
  line L175 (6.2707, -14.2573) -> (4.6986, -14.2573)
  line L176 (4.6986, -14.2573) -> (4.6986, -13.6252)
  line L177 (4.6986, -13.6252) -> (9.8323, -13.6252)
  line L178 (9.8323, -13.6252) -> (9.8323, -14.2573)
  line L179 (9.8323, -14.2573) -> (9.4393, -14.2573)
  spline S174 degree 2 poles (9.4393, -14.2573) (9.654, -14.4923) (9.9377, -15.0677) (9.9377, -15.404) knots 0 0 0 1 2 2 2
  spline S175 degree 2 poles (9.9377, -15.404) (9.9377, -16.0483) (8.9166, -16.7695) (8.0576, -16.7695) knots 0 0 0 1 2 2 2
  spline S176 degree 2 poles (7.9847, -16.1171) (8.6289, -16.1171) (9.338, -15.7079) (9.338, -15.25) knots 0 0 0 1 2 2 2
  spline S177 degree 2 poles (9.338, -15.25) (9.338, -14.9826) (9.0989, -14.4802) (8.9125, -14.2573) knots 0 0 0 1 2 2 2
  line L180 (8.9125, -14.2573) -> (6.7813, -14.2573)
  spline S178 degree 2 poles (6.7813, -14.2573) (6.6637, -14.5045) (6.5746, -14.857) (6.5746, -15.0839) knots 0 0 0 1 2 2 2
  spline S179 degree 2 poles (6.5746, -15.0839) (6.5746, -15.5742) (7.2958, -16.1171) (7.9847, -16.1171) knots 0 0 0 1 2 2 2
  line L181 (9.1556, -19.4154) -> (9.1556, -19.3829)
  spline S180 degree 2 poles (9.1556, -19.3829) (9.1759, -19.31) (9.184, -19.152) (9.184, -19.0426) knots 0 0 0 1 2 2 2
  spline S181 degree 2 poles (9.184, -19.0426) (9.184, -18.7873) (8.9612, -18.2849) (8.7424, -18.058) knots 0 0 0 1 2 2 2
  line L182 (8.7424, -18.058) -> (6.0803, -18.058)
  line L183 (6.0803, -18.058) -> (6.0803, -17.4259)
  line L184 (6.0803, -17.4259) -> (9.8323, -17.4259)
  line L185 (9.8323, -17.4259) -> (9.8323, -18.058)
  line L186 (9.8323, -18.058) -> (9.2731, -18.058)
  spline S182 degree 2 poles (9.2731, -18.058) (9.5811, -18.4024) (9.8323, -18.917) (9.8323, -19.1601) knots 0 0 0 1 2 2 2
  spline S183 degree 2 poles (9.8323, -19.1601) (9.8323, -19.2573) (9.8242, -19.3546) (9.812, -19.4154) knots 0 0 0 1 2 2 2
  line L187 (9.812, -19.4154) -> (9.1556, -19.4154)
  spline S184 degree 2 poles (5.9952, -21.5345) (5.9952, -20.635) (7.0041, -19.6463) (7.936, -19.6463) knots 0 0 0 1 2 2 2
  spline S185 degree 2 poles (7.936, -19.6463) (8.8518, -19.6463) (9.9377, -20.6066) (9.9377, -21.3805) knots 0 0 0 1 2 2 2
  spline S186 degree 2 poles (9.9377, -21.3805) (9.9377, -21.729) (9.7351, -22.2679) (9.5203, -22.4664) knots 0 0 0 1 2 2 2
  spline S187 degree 2 poles (9.5203, -22.4664) (9.3056, -22.669) (8.6856, -22.8837) (8.2359, -22.8837) knots 0 0 0 1 2 2 2
  line L188 (8.2359, -22.8837) -> (7.8915, -22.8837)
  line L189 (7.8915, -22.8837) -> (7.8915, -20.2865)
  spline S188 degree 2 poles (7.8915, -20.2865) (7.2391, -20.2865) (6.5462, -20.9429) (6.5462, -21.5264) knots 0 0 0 1 2 2 2
  spline S189 degree 2 poles (6.5462, -21.5264) (6.5462, -21.733) (6.6394, -22.1342) (6.7124, -22.2962) knots 0 0 0 1 2 2 2
  spline S190 degree 2 poles (6.7124, -22.2962) (6.7934, -22.4664) (6.9352, -22.7014) (7.0001, -22.7784) knots 0 0 0 1 2 2 2
  line L190 (7.0001, -22.7784) -> (7.0001, -22.8149)
  line L191 (7.0001, -22.8149) -> (6.3112, -22.8149)
  spline S191 degree 2 poles (6.3112, -22.8149) (6.2667, -22.7055) (6.137, -22.3732) (6.1005, -22.2436) knots 0 0 0 1 2 2 2
  spline S192 degree 2 poles (6.1005, -22.2436) (6.0479, -22.0612) (5.9952, -21.7614) (5.9952, -21.5345) knots 0 0 0 1 2 2 2
  spline S193 degree 2 poles (8.3736, -22.2679) (8.6289, -22.2598) (9.0017, -22.1544) (9.1273, -22.0531) knots 0 0 0 1 2 2 2
  spline S194 degree 2 poles (9.1273, -22.0531) (9.2691, -21.9437) (9.419, -21.5993) (9.419, -21.344) knots 0 0 0 1 2 2 2
  spline S195 degree 2 poles (9.419, -21.344) (9.419, -21.0928) (9.2691, -20.7403) (9.1232, -20.5944) knots 0 0 0 1 2 2 2
  spline S196 degree 2 poles (9.1232, -20.5944) (8.9733, -20.4526) (8.6127, -20.3068) (8.3736, -20.2865) knots 0 0 0 1 2 2 2
  line L192 (8.3736, -20.2865) -> (8.3736, -22.2679)
  spline S197 degree 2 poles (5.9911, -24.5369) (5.9911, -24.1601) (6.1937, -23.5077) (6.3072, -23.293) knots 0 0 0 1 2 2 2
  line L193 (6.3072, -23.293) -> (7.0163, -23.293)
  line L194 (7.0163, -23.293) -> (7.0163, -23.3254)
  spline S198 degree 2 poles (7.0163, -23.3254) (6.9514, -23.4064) (6.7975, -23.6252) (6.7124, -23.8076) knots 0 0 0 1 2 2 2
  spline S199 degree 2 poles (6.7124, -23.8076) (6.6354, -23.9656) (6.5219, -24.3546) (6.5219, -24.5612) knots 0 0 0 1 2 2 2
  spline S200 degree 2 poles (6.5219, -24.5612) (6.5219, -24.7111) (6.5908, -25.0555) (6.6475, -25.1366) knots 0 0 0 1 2 2 2
  spline S201 degree 2 poles (6.6475, -25.1366) (6.7245, -25.2541) (6.8988, -25.3594) (7.077, -25.3594) knots 0 0 0 1 2 2 2
  spline S202 degree 2 poles (7.077, -25.3594) (7.2999, -25.3594) (7.5308, -25.1163) (7.6078, -24.8043) knots 0 0 0 1 2 2 2
  spline S203 degree 2 poles (7.6078, -24.8043) (7.6362, -24.6828) (7.7172, -24.2938) (7.7618, -24.1277) knots 0 0 0 1 2 2 2
  spline S204 degree 2 poles (7.7618, -24.1277) (7.8874, -23.6982) (8.406, -23.3092) (8.7748, -23.3092) knots 0 0 0 1 2 2 2
  spline S205 degree 2 poles (8.7748, -23.3092) (9.2853, -23.3092) (9.9214, -24.075) (9.9214, -24.7071) knots 0 0 0 1 2 2 2
  spline S206 degree 2 poles (9.9214, -24.7071) (9.9214, -25.0191) (9.7675, -25.6512) (9.65, -25.8659) knots 0 0 0 1 2 2 2
  line L195 (9.65, -25.8659) -> (8.9733, -25.8659)
  line L196 (8.9733, -25.8659) -> (8.9733, -25.8335)
  spline S207 degree 2 poles (8.9733, -25.8335) (9.1678, -25.5904) (9.3907, -24.9988) (9.3907, -24.6949) knots 0 0 0 1 2 2 2
  spline S208 degree 2 poles (9.3907, -24.6949) (9.3907, -24.3829) (9.1273, -23.9534) (8.8639, -23.9534) knots 0 0 0 1 2 2 2
  spline S209 degree 2 poles (8.8639, -23.9534) (8.6248, -23.9534) (8.3939, -24.2087) (8.321, -24.4923) knots 0 0 0 1 2 2 2
  spline S210 degree 2 poles (8.321, -24.4923) (8.2845, -24.6301) (8.2116, -24.9786) (8.167, -25.169) knots 0 0 0 1 2 2 2
  spline S211 degree 2 poles (8.167, -25.169) (8.0616, -25.5823) (7.5795, -26.0037) (7.1621, -26.0037) knots 0 0 0 1 2 2 2
  spline S212 degree 2 poles (7.1621, -26.0037) (6.919, -26.0037) (6.4895, -25.8132) (6.3315, -25.6269) knots 0 0 0 1 2 2 2
  spline S213 degree 2 poles (6.3315, -25.6269) (6.1654, -25.4283) (5.9911, -24.9218) (5.9911, -24.5369) knots 0 0 0 1 2 2 2
  spline S214 degree 2 poles (5.9911, -27.6042) (5.9911, -27.2273) (6.1937, -26.575) (6.3072, -26.3602) knots 0 0 0 1 2 2 2
  line L197 (6.3072, -26.3602) -> (7.0163, -26.3602)
  line L198 (7.0163, -26.3602) -> (7.0163, -26.3927)
  spline S215 degree 2 poles (7.0163, -26.3927) (6.9514, -26.4737) (6.7975, -26.6925) (6.7124, -26.8748) knots 0 0 0 1 2 2 2
  spline S216 degree 2 poles (6.7124, -26.8748) (6.6354, -27.0329) (6.5219, -27.4218) (6.5219, -27.6285) knots 0 0 0 1 2 2 2
  spline S217 degree 2 poles (6.5219, -27.6285) (6.5219, -27.7784) (6.5908, -28.1228) (6.6475, -28.2038) knots 0 0 0 1 2 2 2
  spline S218 degree 2 poles (6.6475, -28.2038) (6.7245, -28.3213) (6.8988, -28.4267) (7.077, -28.4267) knots 0 0 0 1 2 2 2
  spline S219 degree 2 poles (7.077, -28.4267) (7.2999, -28.4267) (7.5308, -28.1836) (7.6078, -27.8716) knots 0 0 0 1 2 2 2
  spline S220 degree 2 poles (7.6078, -27.8716) (7.6362, -27.75) (7.7172, -27.3611) (7.7618, -27.1949) knots 0 0 0 1 2 2 2
  spline S221 degree 2 poles (7.7618, -27.1949) (7.8874, -26.7654) (8.406, -26.3765) (8.7748, -26.3765) knots 0 0 0 1 2 2 2
  spline S222 degree 2 poles (8.7748, -26.3765) (9.2853, -26.3765) (9.9214, -27.1423) (9.9214, -27.7743) knots 0 0 0 1 2 2 2
  spline S223 degree 2 poles (9.9214, -27.7743) (9.9214, -28.0863) (9.7675, -28.7184) (9.65, -28.9332) knots 0 0 0 1 2 2 2
  line L199 (9.65, -28.9332) -> (8.9733, -28.9332)
  line L200 (8.9733, -28.9332) -> (8.9733, -28.9008)
  spline S224 degree 2 poles (8.9733, -28.9008) (9.1678, -28.6577) (9.3907, -28.0661) (9.3907, -27.7622) knots 0 0 0 1 2 2 2
  spline S225 degree 2 poles (9.3907, -27.7622) (9.3907, -27.4502) (9.1273, -27.0207) (8.8639, -27.0207) knots 0 0 0 1 2 2 2
  spline S226 degree 2 poles (8.8639, -27.0207) (8.6248, -27.0207) (8.3939, -27.276) (8.321, -27.5596) knots 0 0 0 1 2 2 2
  spline S227 degree 2 poles (8.321, -27.5596) (8.2845, -27.6974) (8.2116, -28.0458) (8.167, -28.2363) knots 0 0 0 1 2 2 2
  spline S228 degree 2 poles (8.167, -28.2363) (8.0616, -28.6496) (7.5795, -29.0709) (7.1621, -29.0709) knots 0 0 0 1 2 2 2
  spline S229 degree 2 poles (7.1621, -29.0709) (6.919, -29.0709) (6.4895, -28.8805) (6.3315, -28.6941) knots 0 0 0 1 2 2 2
  spline S230 degree 2 poles (6.3315, -28.6941) (6.1654, -28.4956) (5.9911, -27.9891) (5.9911, -27.6042) knots 0 0 0 1 2 2 2
  spline S231 degree 2 poles (5.9952, -31.2873) (5.9952, -30.3878) (7.0041, -29.3991) (7.936, -29.3991) knots 0 0 0 1 2 2 2
  spline S232 degree 2 poles (7.936, -29.3991) (8.8518, -29.3991) (9.9377, -30.3594) (9.9377, -31.1333) knots 0 0 0 1 2 2 2
  spline S233 degree 2 poles (9.9377, -31.1333) (9.9377, -31.4818) (9.7351, -32.0207) (9.5203, -32.2192) knots 0 0 0 1 2 2 2
  spline S234 degree 2 poles (9.5203, -32.2192) (9.3056, -32.4218) (8.6856, -32.6366) (8.2359, -32.6366) knots 0 0 0 1 2 2 2
  line L201 (8.2359, -32.6366) -> (7.8915, -32.6366)
  line L202 (7.8915, -32.6366) -> (7.8915, -30.0393)
  spline S235 degree 2 poles (7.8915, -30.0393) (7.2391, -30.0393) (6.5462, -30.6957) (6.5462, -31.2792) knots 0 0 0 1 2 2 2
  spline S236 degree 2 poles (6.5462, -31.2792) (6.5462, -31.4859) (6.6394, -31.887) (6.7124, -32.0491) knots 0 0 0 1 2 2 2
  spline S237 degree 2 poles (6.7124, -32.0491) (6.7934, -32.2192) (6.9352, -32.4543) (7.0001, -32.5312) knots 0 0 0 1 2 2 2
  line L203 (7.0001, -32.5312) -> (7.0001, -32.5677)
  line L204 (7.0001, -32.5677) -> (6.3112, -32.5677)
  spline S238 degree 2 poles (6.3112, -32.5677) (6.2667, -32.4583) (6.137, -32.126) (6.1005, -31.9964) knots 0 0 0 1 2 2 2
  spline S239 degree 2 poles (6.1005, -31.9964) (6.0479, -31.8141) (5.9952, -31.5142) (5.9952, -31.2873) knots 0 0 0 1 2 2 2
  spline S240 degree 2 poles (8.3736, -32.0207) (8.6289, -32.0126) (9.0017, -31.9072) (9.1273, -31.806) knots 0 0 0 1 2 2 2
  spline S241 degree 2 poles (9.1273, -31.806) (9.2691, -31.6966) (9.419, -31.3521) (9.419, -31.0969) knots 0 0 0 1 2 2 2
  spline S242 degree 2 poles (9.419, -31.0969) (9.419, -30.8457) (9.2691, -30.4931) (9.1232, -30.3473) knots 0 0 0 1 2 2 2
  spline S243 degree 2 poles (9.1232, -30.3473) (8.9733, -30.2055) (8.6127, -30.0596) (8.3736, -30.0393) knots 0 0 0 1 2 2 2
  line L205 (8.3736, -30.0393) -> (8.3736, -32.0207)
  line L206 (6.0803, -36.2225) -> (6.0803, -35.5904)
  line L207 (6.0803, -35.5904) -> (8.2197, -35.5904)
  spline S244 degree 2 poles (8.2197, -35.5904) (8.479, -35.5904) (8.9247, -35.5418) (9.0584, -35.4688) knots 0 0 0 1 2 2 2
  spline S245 degree 2 poles (9.0584, -35.4688) (9.2002, -35.3919) (9.338, -35.1163) (9.338, -34.8813) knots 0 0 0 1 2 2 2
  spline S246 degree 2 poles (9.338, -34.8813) (9.338, -34.6463) (9.0868, -34.1479) (8.8842, -33.9089) knots 0 0 0 1 2 2 2
  line L208 (8.8842, -33.9089) -> (6.0803, -33.9089)
  line L209 (6.0803, -33.9089) -> (6.0803, -33.2768)
  line L210 (6.0803, -33.2768) -> (9.8323, -33.2768)
  line L211 (9.8323, -33.2768) -> (9.8323, -33.9089)
  line L212 (9.8323, -33.9089) -> (9.415, -33.9089)
  spline S247 degree 2 poles (9.415, -33.9089) (9.6702, -34.1925) (9.9377, -34.7395) (9.9377, -35.0474) knots 0 0 0 1 2 2 2
  spline S248 degree 2 poles (9.9377, -35.0474) (9.9377, -35.5985) (9.2083, -36.2225) (8.5154, -36.2225) knots 0 0 0 1 2 2 2
  line L213 (8.5154, -36.2225) -> (6.0803, -36.2225)
  point P0 (0, 0)
  dimension "d1" = 2
  dimension "d2" = 2
  dimension "d3" = 2
  dimension "d4" = 2
  dimension "d5" = 24
  dimension "d6" = 90
  dimension "d7" = 3.5
  dimension "d8" = 3
  dimension "d9" = 3
  dimension "d10" = 3.5
  dimension "d11" = 3
  dimension "d12" = 3
  constraints: 10 end point, 4 centre point, 2 midpoint, 2 parallel, 2 symmetric about line, 1 horizontal, 1 perpendicular, 4 other
  measures "d1" distance between parallel lines of L0 L7
  measures "d2" distance between parallel lines of L2 L5
  measures "d3" distance between parallel lines of L3 L4
  measures "d4" distance between parallel lines of L1 L6
  measures "d5" distance of L1.end L2.end
  measures "d6" distance of L2.end L0.start
  measures "d7" diameter of A0
  measures "d8" distance from line of L3 A0.centre
  measures "d9" distance from line of L0 A0.centre
  measures "d10" diameter of A1
  measures "d11" distance from line of L1 A1.centre
  measures "d12" distance from line of L0 A1.centre
extrude "Extrusion1" add sketch "Sketch1" against normal blind 3 contours L3 L2 L1 L0 | S0 S1 L9 L10 L11 S2 S3 | S7 S6 L14 L13 L12 S5 S4 | L15 L16 L17 L18 L19 L20 L21 L22 L23 L24 L25 L26 | L27 L28 L29 L30 L31 L32 L33 L34 L35 L36 | S8 S9 S10 S11 S12 S13 S14 L37 L38 S15 S16 S17 S18 S19 | S26 S25 S24 S23 S22 S21 S20 | L39 L40 L41 L42 L43 L44 S27 L45 L46 L47 L48 | S28 S29 S30 S31 S32 S33 S34 L49 L50 S35 S36 S37 S38 S39 | S46 S45 S44 S43 S42 S41 S40 | L51 L52 L53 L54 L55 L56 L57 L58 L59 L60 | L61 L62 L63 L64 | S47 S48 S49 S50 S51 S52 L65 S53 S54 S55 L66 L67 S56 S57 S58 L68 L69 L70 | S62 S61 S60 S59 L71 | L72 S63 S64 S65 S66 L73 L74 L75 S67 S68 S69 L76 L77 L78 L79 L80 S70 S71 S72 S73 S74 L81 L82 | L83 S75 S76 S77 S78 L84 L85 L86 S79 S80 S81 L87 L88 L89 L90 L91 S82 S83 S84 S85 S86 L92 L93 | S87 S88 S89 S90 L94 L95 S91 S92 S93 L96 L97 S94 S95 | L98 S99 S98 S97 S96 | L99 L100 L101 L102 L103 L104 L105 L106 L107 L108 L109 L110 | S100 S101 S102 S103 S104 S105 L111 S106 S107 S108 L112 L113 S109 S110 S111 L114 L115 L116 | S115 S114 S113 S112 L117 | S116 L118 L119 S117 S118 S119 S120 S121 S122 S123 S124 S125 L120 L121 S126 S127 S128 S129 S130 S131 S132 | S133 L122 L123 L124 L125 L126 L127 L128 L129 L130 L131 L132 S134 S135 S136 L133 L134 S137 | S138 S139 S140 S141 L135 L136 S142 S143 S144 L137 L138 S145 S146 | L139 S150 S149 S148 S147 | L140 S151 S152 L141 L142 L143 L144 L145 S153 S154 L146 | L147 L148 L149 L150 L151 L152 L153 L154 L155 L156 L157 L158 | L159 L160 L161 L162 L163 L164 L165 L166 L167 L168 L169 L170 | S155 L171 L172 S156 S157 S158 S159 S160 S161 S162 S163 S164 L173 L174 S165 S166 S167 S168 S169 S170 S171 | S172 S173 L175 L176 L177 L178 L179 S174 S175 | S179 S178 L180 S177 S176 | L181 S180 S181 L182 L183 L184 L185 L186 S182 S183 L187 | S184 S185 S186 S187 L188 L189 S188 S189 S190 L190 L191 S191 S192 | L192 S196 S195 S194 S193 | S197 L193 L194 S198 S199 S200 S201 S202 S203 S204 S205 S206 L195 L196 S207 S208 S209 S210 S211 S212 S213 | S214 L197 L198 S215 S216 S217 S218 S219 S220 S221 S222 S223 L199 L200 S224 S225 S226 S227 S228 S229 S230 | S231 S232 S233 S234 L201 L202 S235 S236 S237 L203 L204 S238 S239 | L205 S243 S242 S241 S240 | L206 L207 S244 S245 S246 L208 L209 L210 L211 L212 S247 S248 L213
extrude "Extrusion2" add sketch "Sketch1" along normal blind 1 contours S0 S1 L9 L10 L11 S2 S3 | L15 L16 L17 L18 L19 L20 L21 L22 L23 L24 L25 L26 | L27 L28 L29 L30 L31 L32 L33 L34 L35 L36 | S8 S9 S10 S11 S12 S13 S14 L37 L38 S15 S16 S17 S18 S19 | L39 L40 L41 L42 L43 L44 S27 L45 L46 L47 L48 | S28 S29 S30 S31 S32 S33 S34 L49 L50 S35 S36 S37 S38 S39 | L51 L52 L53 L54 L55 L56 L57 L58 L59 L60 | L61 L62 L63 L64 | S47 S48 S49 S50 S51 S52 L65 S53 S54 S55 L66 L67 S56 S57 S58 L68 L69 L70 | L72 S63 S64 S65 S66 L73 L74 L75 S67 S68 S69 L76 L77 L78 L79 L80 S70 S71 S72 S73 S74 L81 L82 | L83 S75 S76 S77 S78 L84 L85 L86 S79 S80 S81 L87 L88 L89 L90 L91 S82 S83 S84 S85 S86 L92 L93 | S87 S88 S89 S90 L94 L95 S91 S92 S93 L96 L97 S94 S95 | L99 L100 L101 L102 L103 L104 L105 L106 L107 L108 L109 L110 | S100 S101 S102 S103 S104 S105 L111 S106 S107 S108 L112 L113 S109 S110 S111 L114 L115 L116 | S116 L118 L119 S117 S118 S119 S120 S121 S122 S123 S124 S125 L120 L121 S126 S127 S128 S129 S130 S131 S132 | S133 L122 L123 L124 L125 L126 L127 L128 L129 L130 L131 L132 S134 S135 S136 L133 L134 S137 | S138 S139 S140 S141 L135 L136 S142 S143 S144 L137 L138 S145 S146 | L140 S151 S152 L141 L142 L143 L144 L145 S153 S154 L146 | L147 L148 L149 L150 L151 L152 L153 L154 L155 L156 L157 L158 | L159 L160 L161 L162 L163 L164 L165 L166 L167 L168 L169 L170 | S155 L171 L172 S156 S157 S158 S159 S160 S161 S162 S163 S164 L173 L174 S165 S166 S167 S168 S169 S170 S171 | S172 S173 L175 L176 L177 L178 L179 S174 S175 | L181 S180 S181 L182 L183 L184 L185 L186 S182 S183 L187 | S184 S185 S186 S187 L188 L189 S188 S189 S190 L190 L191 S191 S192 | S197 L193 L194 S198 S199 S200 S201 S202 S203 S204 S205 S206 L195 L196 S207 S208 S209 S210 S211 S212 S213 | S214 L197 L198 S215 S216 S217 S218 S219 S220 S221 S222 S223 L199 L200 S224 S225 S226 S227 S228 S229 S230 | S231 S232 S233 S234 L201 L202 S235 S236 S237 L203 L204 S238 S239 | L206 L207 S244 S245 S246 L208 L209 L210 L211 L212 S247 S248 L213
fillet "Fillet1" radius 3 4 edges at (-0.0563, -1.5, -43.5179) (-24.0563, -1.5, -43.5179) (-24.0563, -1.5, 46.4821) (-0.0563, -1.5, 46.4821)
body "Solid1"
